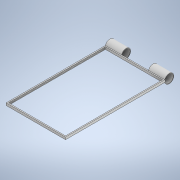
# Autodesk Inventor part: вращалка
Saved by Autodesk Inventor 2022.4 (Build 264492010, 492A)
## iProperties
Created: 2023-02-20
Part Number: вращалка
Material: Типовые
Document SubType Name: Modeling
Designer: artyo
Density: 1 g/cm^3
Appearance: По умолчанию
Author: artyo
Autodesk Inventor part; units mm, degrees
ref_plane "YZ Plane" through (0, 0, 0) normal (1, 0, 0) x (0, 1, 0)
ref_plane "XZ Plane" through (0, 0, 0) normal (0, 1, 0) x (-1, 0, 0)
sketch "Эскиз1" plane through (0, 0, 0) normal (1, 0, 0) x (0, 1, 0)
  circle A0 centre (0, 0) radius 7.5
  circle A1 centre (0, 0) radius 8.5
  dimension "d0" = 15
  dimension "d1" = 17
  constraints: 2 centre point, 2 coincident
  measures "d0" diameter of A0
  measures "d1" diameter of A1
extrude "Выдавливание1" add sketch "Эскиз1" along normal blind 30
ref_plane "РабПлоскость1" through (80, 0, 0) normal (1, 0, 0) x (0, 0, -1)
sketch "Эскиз2" plane through (80, 0, 0) normal (1, 0, 0) x (0, 0, -1)
  circle A0 centre (0, 0) radius 8.5
  circle A1 centre (0, 0) radius 7.5
  dimension "d5" = 17
  dimension "d6" = 15
  constraints: 2 centre point, 2 coincident
  measures "d5" diameter of A0
  measures "d6" diameter of A1
extrude "Выдавливание2" add sketch "Эскиз2" along normal blind 30
sketch "Эскиз3" plane through (0, 0, 0) normal (-1, 0, 0) x (0, 0, 1)
  circle A0 centre (0, 0) radius 7.5 projected
  line L0 (-7.5, 0) -> (7.5, 0)
  circle A1 centre (0, 0) radius 8.5 projected
  circle A2 centre (0, 0) radius 7.5 projected
  circle A3 centre (0, 0) radius 8.5 projected
  line L1 (8.2203, -2.1625) -> (12.2203, -2.1625)
  line L2 (8.2203, 2.1625) -> (12.2203, 2.1625)
  line L3 (12.2203, -2.1625) -> (12.2203, 2.1625)
  arc A4 (8.2203, -2.1625) -> (8.2203, 2.1625) centre (0, 0) ccw
  dimension "d9" = 4
  constraints: 8 end point, 4 point on circle, 2 horizontal, 2 symmetric about line, 1 centre point, 1 perpendicular, 3 other
  measures "d9" distance of L1.start L1.end
extrude "Выдавливание3" add sketch "Эскиз3" against normal blind 110 contours A1 L2 L3 L1
sketch "Эскиз4" plane through (0, -2.1625, 12.2203) normal (0, 0, 1) x (1, 0, 0)
  line L0 (0, 4.325) -> (30, 4.325) projected
  line L1 (0, 0) -> (110, 0) projected
  line L2 (0, 4.325) -> (110, 4.325)
  line L3 (110, 4.325) -> (110, 0)
  line L4 (110, 0) -> (0, 0)
  line L5 (0, 0) -> (0, 4.325)
  line L6 (109, 1) -> (1, 1)
  line L7 (1, 1) -> (1, 3.325)
  line L8 (1, 3.325) -> (109, 3.325)
  line L9 (109, 3.325) -> (109, 1)
  line L10 (109, 1) -> (1, 3.325) construction
  line L11 (1, 1) -> (109, 3.325) construction
  line L12 (0, 4.325) -> (110, 4.325) projected
  line L13 (110, 0) -> (0, 0)
  line L14 (0, 0) -> (0, 4.325)
  line L15 (0, 4.325) -> (110, 4.325)
  line L16 (110, 4.325) -> (110, 0)
  line L17 (110, 0) -> (0, 4.325) construction
  line L18 (0, 0) -> (110, 4.325) construction
  point P0 (0, 2.1625)
  point P1 (55, 2.1625)
  point P2 (55, 2.1625)
  dimension "d12" = 108
  dimension "d13" = 2.325
  constraints: 32 end point, 6 parallel, 5 midpoint, 3 horizontal, 3 perpendicular
  measures "d12" distance of L7.end L8.end
  measures "d13" distance of L6.end L7.end
extrude "Выдавливание4" add sketch "Эскиз4" along normal blind 180 contours L0 L2 L3 L1 L5 | L6 L7 L8 L9
sketch "Эскиз5" plane through (30, 2.1625, 8.2203) normal (0, 1, 0) x (1, 0, 0)
  line L0 (80, -184) -> (-30, -184) projected
  line L1 (25, -184) -> (25, -92)
  line L2 (-28, -2) -> (78, -2)
  line L3 (78, -2) -> (78, -182)
  line L4 (78, -182) -> (-28, -182)
  line L5 (-28, -182) -> (-28, -2)
  line L6 (-28, -2) -> (78, -182) construction
  line L7 (78, -2) -> (-28, -182) construction
  point P0 (-30, 8.2203)
  dimension "d16" = 92
  dimension "d17" = 106
  dimension "d18" = 180
  constraints: 14 end point, 3 midpoint, 2 parallel, 1 horizontal, 1 perpendicular, 1 vertical
  measures "d16" distance of L1.start L1.end
  measures "d17" distance of L3.end L4.end
  measures "d18" distance of L2.end L3.end
extrude "Выдавливание5" cut sketch "Эскиз5" against normal blind 180
sketch "Эскиз6" plane through (108, 2.1625, 10.2203) normal (-1, 0, 0) x (0, 0, 1)
  line L0 (0, 0) -> (180, 0) projected
  line L1 (0, 0) -> (0, -1)
  line L2 (0, 0) -> (0, -4.325) projected
  line L3 (0, -1) -> (180, -1)
  line L4 (180, -1) -> (180, -3.325)
  line L5 (180, -3.325) -> (0, -3.325)
  line L6 (0, -3.325) -> (0, -1)
  point P0 (-10.2203, -2.1625)
  point P1 (0, -3.325)
  dimension "d21" = 1
  dimension "d22" = 2.325
  constraints: 10 end point, 4 perpendicular, 2 point on line
  measures "d21" distance of L0.start L1.end
  measures "d22" distance of L3.end L4.end
extrude "Выдавливание6" cut sketch "Эскиз6" along normal blind 107 and the other way blind 1
